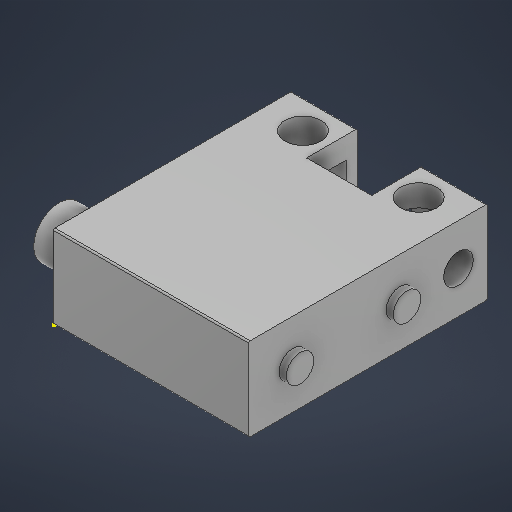
# Autodesk Inventor part: MS 1.5A Servo
Saved by Autodesk Inventor 2026.1 (Build 301233020, 233B)
## iProperties
Created: 2025-10-17
Part Number: MS 1.5A Servo
Material: Generic
Document SubType Name: Modeling
Designer: MP2BD9BR
Density: 1 g/cm^3
Appearance: Smooth - Medium Gray
Author: MP2BD9BR
Autodesk Inventor part; units mm, degrees
ref_plane "YZ Plane" through (0, 0, 0) normal (1, 0, 0) x (0, 1, 0)
ref_plane "XZ Plane" through (0, 0, 0) normal (0, 1, 0) x (-1, 0, 0)
ref_plane "XY Plane" through (0, 0, 0) normal (0, 0, 1) x (1, 0, 0)
sketch "Sketch1" plane through (0, 0, 0) normal (0, 1, 0) x (-1, 0, 0)
  line L0 (0, 0) -> (-27, 0)
  line L1 (-27, 0) -> (-27, -33)
  line L2 (-27, -33) -> (0, -33)
  line L3 (0, -33) -> (0, 0)
  dimension "d0" = 33
  dimension "d1" = 27
  constraints: 8 end point, 2 parallel, 1 horizontal, 1 perpendicular
  measures "d0" distance between parallel lines of L0 L2
  measures "d1" distance between parallel lines of L1 L3
extrude "Extrusion1" add sketch "Sketch1" along normal blind 11.5
sketch "Sketch2" plane through (0, 0, -33) normal (-1, 0, 0) x (0, 0, 1)
  circle A0 centre (27.25, 5.75) radius 3.5
  line L0 (0, 11.5) -> (33, 11.5) projected
  line L1 (33, 0) -> (33, 11.5) projected
  dimension "d4" = 7
  dimension "d5" = 5.75
  dimension "d6" = 5.75
  constraints: 1 centre point
  measures "d4" diameter of A0
  measures "d5" distance from line of L0 A0.centre
  measures "d6" distance from line of L1 A0.centre
extrude "Extrusion2" add sketch "Sketch2" along normal blind 5
sketch "Sketch3" plane through (0, 11.5, 0) normal (0, 1, 0) x (1, 0, 0)
  line L0 (27, 33) -> (0, 33) projected
  line L1 (9, 33) -> (18, 33)
  line L2 (18, 33) -> (18, 26)
  line L3 (18, 26) -> (9, 26)
  line L4 (9, 26) -> (9, 33)
  line L5 (27, 0) -> (27, 33) projected
  point P0 (0, 0)
  dimension "d9" = 9
  dimension "d10" = 9
  dimension "d11" = 7
  constraints: 8 end point, 2 parallel, 1 horizontal, 1 perpendicular, 1 point on line
  measures "d9" distance between parallel lines of L2 L4
  measures "d10" distance between parallel lines of L5 L2
  measures "d11" distance between parallel lines of L0 L3
extrude "Extrusion3" cut sketch "Sketch3" against normal blind 9
sketch "Sketch4" plane through (0, 11.5, 0) normal (0, 1, 0) x (1, 0, 0)
  circle A0 centre (5.5, 29) radius 2.5
  circle A1 centre (21.5, 29) radius 2.5
  line L0 (9, 33) -> (18, 33) construction
  line L1 (13.5, 33) -> (13.5, 0) construction
  line L2 (0, 0) -> (27, 0) construction
  line L3 (9, 33) -> (0, 33) construction
  dimension "d14" = 5
  dimension "d15" = 5
  dimension "d16" = 16
  dimension "d17" = 8
  dimension "d18" = 4
  dimension "d19" = 8
  constraints: 2 centre point, 2 end point, 2 midpoint
  measures "d14" diameter of A0
  measures "d15" diameter of A1
  measures "d16" distance of A1.centre A0.centre
  measures "d17" distance from line of L1 A0.centre
  measures "d18" distance from line of L3 A0.centre
  measures "d19" distance from line of L1 A1.centre
extrude "Extrusion4" cut sketch "Sketch4" against normal blind 15
sketch "Sketch5" plane through (0, 0, -33) normal (-1, 0, 0) x (0, 0, 1)
  circle A0 centre (4, 5.75) radius 2.05
  line L0 (0, 0) -> (0, 11.5) projected
  line L1 (33, 0) -> (33, 11.5) construction
  line L2 (33, 5.75) -> (0, 5.75) construction
  dimension "d22" = 4.1
  dimension "d23" = 4
  dimension "d24" = 0
  constraints: 2 end point, 2 midpoint, 1 centre point
  measures "d22" diameter of A0
  measures "d23" distance from line of L0 A0.centre
  measures "d24" distance from line of L2 A0.centre
extrude "Extrusion5" cut sketch "Sketch5" against normal blind 31.75
sketch "Sketch6" plane through (0, 0, 0) normal (0, -1, 0) x (1, 0, 0)
  point P0 (0, 0)
sketch "Sketch12" plane through (27, 0, -33) normal (1, 0, 0) x (0, 0, -1)
  line L0 (-33, 0) -> (0, 0) projected
  line L1 (-8.9949, 0) -> (-8.9949, 11.5163)
  point P0 (-32.75, 0)
  constraints: 2 end point, 1 point on line, 1 vertical
sketch "Sketch13" plane through (0, 0, -33) normal (-1, 0, 0) x (0, 0, 1)
  line L0 (0, 0) -> (33, 0) projected
  line L1 (9, 0) -> (9, 11.5008)
  point P0 (32.75, 0)
  constraints: 2 end point, 1 point on line, 1 vertical
sketch "Sketch16" plane through (0, 11.5, 0) normal (0, 1, 0) x (1, 0, 0)
  line L0 (0, 33) -> (0, 0) projected
  line L1 (27, 0) -> (27, 33) projected
  line L2 (11, 24) -> (11, 0)
  line L3 (21, 0) -> (21, 24)
  line L4 (0, 24) -> (11, 24)
  line L5 (21, 24) -> (27, 24)
  constraints: 8 end point, 2 horizontal, 2 perpendicular, 2 point on line, 1 vertical
sketch "Sketch17" plane through (0, 0, 0) normal (0, 0, 1) x (1, 0, 0)
  line L0 (0, 11.5) -> (27, 11.5) projected
  line L1 (11, 11.5) -> (11, 0)
  line L2 (21, 0) -> (21, 11.5)
  point P0 (0, 0)
  constraints: 4 end point, 1 point on line, 1 vertical
sketch "Sketch18" plane through (0, 0, 0) normal (0, -1, 0) x (1, 0, 0)
  line L0 (27, 0) -> (27, -33) projected
  line L1 (0, 0) -> (27, 0) projected
  line L2 (21, 0) -> (21, -24)
  line L3 (11, 0) -> (11, -24)
  line L4 (27, -24) -> (21, -24)
  line L5 (11, -24) -> (0, -24)
  line L6 (27, -24) -> (27, -33)
  line L7 (0, -33) -> (0, 0) projected
  line L8 (0, -24) -> (0, -33)
  line L9 (0, -33) -> (27, -33)
  line L10 (21, 0) -> (11, 0)
  constraints: 16 end point, 5 perpendicular, 3 collinear, 3 point on line, 2 horizontal
fillet "Fillet5" radius 0.2 1 edges at (13.5, 11.5, 0)
fillet "Fillet7" radius 0.2 4 edges at (4.5, 11.5, -33) (22.5, 11.5, -33) (13.5, 0, -33) (13.5, 0, 0)
sketch "Sketch20" plane through (9, 2.5, -26) normal (1, 0, 0) x (0, 0, -1)
  line L0 (0, 6) -> (7, 6)
  line L1 (7, 8.8) -> (7, 0) projected
  line L2 (0, 6) -> (7, 6) construction
  line L3 (0, 9) -> (6.8, 9) projected
  line L4 (5.2368, 1.5) -> (10, 1.5) construction
  line L5 (0, 1.5) -> (0, 6)
  line L6 (0, 9) -> (0, 0) projected
  line L7 (0, 0) -> (0, 1)
  line L8 (0, 1) -> (5.2368, 1)
  line L9 (7, 6) -> (5.5, 6)
  line L10 (5.5, 6) -> (5.5, 1)
  line L11 (5.5, 1) -> (5.2368, 1)
  point P0 (-26, -2.5)
  dimension "d41" = 0
  dimension "d43" = 1
  dimension "d44" = 1.5
  constraints: 18 end point, 3 point on line, 2 collinear, 2 horizontal, 2 perpendicular
  measures "d41" distance between parallel lines of L0 L2
  measures "d43" distance of L6.end L7.end
  measures "d44" distance of L2.end L9.end
extrude "Extrusion6" cut sketch "Sketch20" against normal blind 3
sketch "Sketch21" plane through (18, 2.5, -26) normal (-1, 0, 0) x (0, 0, 1)
  line L0 (-7, 0) -> (0, 0) projected
  line L1 (0, 0) -> (0, 1)
  line L2 (0, 9) -> (0, 0) projected
  line L3 (0, 1) -> (-5.5, 1)
  line L4 (0, 9) -> (0, 6)
  line L5 (0, 6) -> (-5.5, 6)
  line L6 (-5.5, 6) -> (-5.5, 1)
  point P0 (26, -2.5)
  dimension "d47" = 1
  dimension "d48" = 5.5
  dimension "d49" = 3
  dimension "d50" = 5.5
  constraints: 10 end point, 2 perpendicular, 2 point on line
  measures "d47" distance of L0.end L1.end
  measures "d48" distance of L1.end L3.end
  measures "d49" distance of L2.start L4.end
  measures "d50" distance of L4.end L5.end
extrude "Extrusion7" cut sketch "Sketch21" against normal blind 3
sketch "Sketch22" plane through (0, 0, -32.8) normal (-1, 0, 0) x (0, 0, 1)
  point P0 (32.8, 0)
sketch "Sketch23" plane through (0, 0, -32.8) normal (-1, 0, 0) x (0, 0, 1)
  line L0 (32.8, 0.2) -> (32.8, 11.3) projected
  line L1 (32.8, 5.75) -> (56.8, 5.75) construction
  circle A0 centre (11.9, 5.75) radius 1.9
  point P0 (32.8, 0)
  constraints: 2 end point, 1 centre point, 1 horizontal, 1 midpoint
extrude "Extrusion8" add sketch "Sketch23" along normal blind 1
sketch "Sketch24" plane through (27, 0, -0.2) normal (1, 0, 0) x (0, 0, -1)
  line L0 (-0.2, 0.2) -> (-0.2, 11.3) projected
  circle A0 centre (20.7, 5.75) radius 1.9
  circle A1 centre (5.9, 5.75) radius 1.9
  point P0 (-0.2, 0)
  constraints: 2 centre point
extrude "Extrusion9" add sketch "Sketch24" along normal blind 1
body "Solid1"
